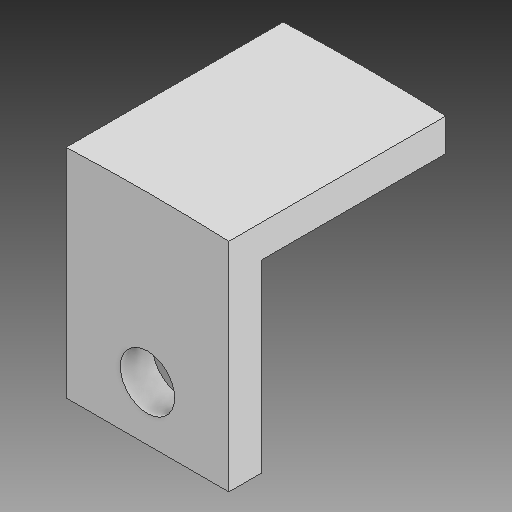
# Autodesk Inventor part: WinkelVentilator
Saved by Autodesk Inventor 2021 (Build 250183000, 183)
## iProperties
Created: 2021-08-26
Part Number: WinkelVentilator
Material: Generisch
Document SubType Name: Modeling
Designer: lukas
Density: 1 g/cm^3
Appearance: Vorgabe
Stock Number: Winkel Ventilator
Author: lukas
Autodesk Inventor part; units mm, degrees
ref_plane "YZ Plane" through (0, 0, 0) normal (1, 0, 0) x (0, 1, 0)
ref_plane "XZ Plane" through (0, 0, 0) normal (0, 1, 0) x (-1, 0, 0)
ref_plane "XY Plane" through (0, 0, 0) normal (0, 0, 1) x (1, 0, 0)
sketch "Skizze5" plane through (0, 0, 0) normal (0, 0, 1) x (1, 0, 0)
  line L0 (-257.6, 0) -> (257.6, 0) projected
  line L1 (0, -257.6) -> (0, 257.6) projected
  circle A0 centre (0, 0) radius 184
  line L2 (0, 0) -> (0, 184)
  line L3 (-7.5, 183.8471) -> (7.5, 183.8471)
  line L4 (-7.5, 183.8471) -> (-7.5, 163.8471)
  line L5 (7.5, 183.8471) -> (7.5, 163.8471)
  line L6 (-7.5, 163.8471) -> (7.5, 163.8471)
  dimension "d14" = 368
  dimension "d15" = 15
  dimension "d16" = 20
  dimension "d17" = 20
  constraints: 10 end point, 3 point on circle, 2 vertical, 1 centre point, 1 coincident, 1 horizontal, 1 point on line
  measures "d14" diameter of A0
  measures "d15" distance of L3.start L3.end
  measures "d16" distance of L3.start L4.end
  measures "d17" distance of L3.end L5.end
extrude "Extrusion3" add sketch "Skizze5" along normal blind 3 contours L6 L4 L3 L1 | L1 L3 L5 L6 | L3 L1 A0 | A0 L1 L3
sketch "Skizze6" plane through (0, 0, 0) normal (0, 0, -1) x (-1, 0, 0)
  line L0 (-7.5, 163.8471) -> (-7.5, 183.8471) projected
  arc A0 (7.5, 183.8471) -> (-7.5, 183.8471) centre (0, 0) ccw projected
  arc A1 (-7.5, 183.8471) -> (0, 184) centre (0, 0) ccw
  line L1 (-7.5, 183.8471) -> (7.5, 183.8471)
  line L2 (7.5, 183.8471) -> (7.5, 180.8471)
  line L3 (7.5, 180.8471) -> (-7.5, 180.8471)
  line L4 (-7.5, 180.8471) -> (-7.5, 183.8471)
  point P0 (7.5, 183.8471)
  point P1 (-7.5, 180.8471)
  dimension "d20" = 3
  constraints: 8 end point, 4 point on circle, 2 parallel, 1 centre point, 1 horizontal, 1 perpendicular
  measures "d20" distance of L1.end L2.end
extrude "Extrusion4" add sketch "Skizze6" along normal blind 17 contours L0 L1 L2 L3 | A0 L1
sketch "Skizze7" plane through (0, 0, 3) normal (0, 0, 1) x (1, 0, 0)
  line L0 (-7.5, 163.8471) -> (7.5, 163.8471) projected
  circle A0 centre (0, 168.8471) radius 2.5
  point P0 (0, 0)
  dimension "d23" = 5
  dimension "d24" = 5
  constraints: 1 centre point, 1 coincident
  measures "d23" distance from line of point (0, 168.847) L0
  measures "d24" diameter of A0
extrude "Extrusion5" cut sketch "Skizze7" against normal blind 17
